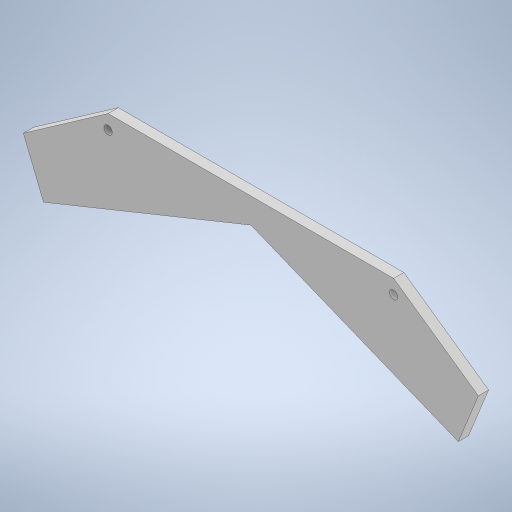
# Autodesk Inventor part: zaver
Saved by Autodesk Inventor 2024 (Build 280153000, 153)
## iProperties
Created: 2024-03-06
Part Number: zaver
Material: Všeobecné
Document SubType Name: Modeling
Designer: Game
Density: 1 g/cm^3
Appearance: Výchozí
Author: Game
Autodesk Inventor part; units mm, degrees
ref_plane "YZ Plane" through (0, 0, 0) normal (1, 0, 0) x (0, 1, 0)
ref_plane "XZ Plane" through (0, 0, 0) normal (0, 1, 0) x (-1, 0, 0)
ref_plane "XY Plane" through (0, 0, 0) normal (0, 0, 1) x (1, 0, 0)
sketch "Náčrt1" plane through (0, 0, 0) normal (0, 0, 1) x (1, 0, 0)
  line L0 (70, 10) -> (-70, 10)
  line L1 (70, 10) -> (136.3513, -36.4597)
  line L2 (70, 10) -> (151, 10) construction
  line L3 (136.3513, -36.4597) -> (124.8798, -52.8427)
  line L4 (-70, 10) -> (-136.3513, -36.4597)
  line L5 (-70, 10) -> (11, 10) construction
  line L6 (-136.3513, -36.4597) -> (-124.8798, -52.8427)
  line L7 (0, 10) -> (0, -2.363)
  line L8 (-124.8798, -52.8427) -> (0, -2.363)
  line L9 (124.8798, -52.8427) -> (0, -2.363)
  point P0 (0, 0)
  dimension "d2" = 140
  dimension "d3" = 81
  dimension "d4" = 35
  dimension "d5" = 20
  dimension "d6" = 81
  dimension "d7" = 145
  dimension "d8" = 20
  dimension "d9" = 12.363
  constraints: 20 end point, 3 perpendicular, 2 equal length, 2 horizontal, 1 point on line
  measures "d2" distance of L0.start L0.end
  measures "d3" distance of L0.start L1.end
  measures "d4" angle of L1 L2
  measures "d5" distance of L1.end L3.end
  measures "d6" distance of L0.end L4.end
  measures "d7" angle of L4 L5
  measures "d8" distance of L4.end L6.end
  measures "d9" distance of L7.start L7.end
extrude "Vysunutí1" add sketch "Náčrt1" along normal blind 5
sketch "Náčrt2" plane through (0, 0, 5) normal (0, 0, 1) x (1, 0, 0)
  line L0 (-136.3513, -36.4597) -> (-124.8798, -52.8427) projected
  line L1 (-124.8798, -52.8427) -> (-101.7018, -43.4736)
  line L2 (-124.8798, -52.8427) -> (0, -2.363) projected
  line L3 (-101.7018, -43.4736) -> (-111.5553, -19.0974)
  line L4 (-70, 10) -> (-136.3513, -36.4597) projected
  line L5 (-136.3513, -36.4597) -> (-124.8798, -52.8427)
  line L6 (0, -2.363) -> (124.8798, -52.8427) projected
  line L7 (124.8798, -52.8427) -> (101.7018, -43.4736)
  line L8 (101.7018, -43.4736) -> (111.5553, -19.0974)
  line L9 (136.3513, -36.4597) -> (70, 10) projected
  line L10 (136.3513, -36.4597) -> (111.5553, -19.0974)
  line L11 (124.8798, -52.8427) -> (136.3513, -36.4597) projected
  line L12 (124.8798, -52.8427) -> (136.3513, -36.4597)
  point P0 (0, 0)
  dimension "d12" = 25
  dimension "d13" = 25
  constraints: 14 end point, 4 point on line, 3 perpendicular, 2 collinear
  measures "d12" distance of L0.end L1.end
  measures "d13" distance of L6.end L7.end
extrude "Vysunutí2" cut sketch "Náčrt2" against normal blind 5
sketch "Náčrt4" plane through (0, 0, 5) normal (0, 0, 1) x (1, 0, 0)
  line L0 (-70, 10) -> (-111.5553, -19.0974) projected
  line L1 (-70, 10) -> (-70, 3.045)
  circle A0 centre (-70, 3.045) radius 2
  line L2 (111.5553, -19.0974) -> (70, 10) projected
  line L3 (70, 10) -> (70, 3.045)
  circle A1 centre (70, 3.045) radius 2
  point P0 (0, 0)
  dimension "d16" = 6.955
  dimension "d17" = 4
  dimension "d18" = 6.955
  dimension "d19" = 4
  constraints: 4 end point, 2 centre point, 2 coincident, 2 vertical
  measures "d16" distance of L0.start L1.end
  measures "d17" diameter of A0
  measures "d18" distance of L2.end L3.end
  measures "d19" diameter of A1
extrude "Vysunutí3" cut sketch "Náčrt4" against normal blind 5
